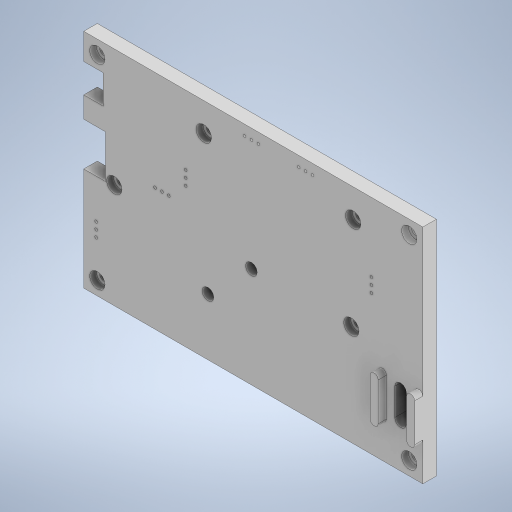
# Autodesk Inventor part: base_main
Saved by Autodesk Inventor 2024.2 (Build 282272000, 272)
## iProperties
Created: 2021-12-13
Part Number: base_main
Material: Generic
Document SubType Name: Modeling
Designer: magoo
Density: 1 g/cm^3
Appearance: Default
Description: 3D printing model
Author: magoo
Autodesk Inventor part; units mm, degrees
ref_plane "YZ Plane" through (0, 0, 0) normal (1, 0, 0) x (0, 1, 0)
ref_plane "XZ Plane" through (0, 0, 0) normal (0, 1, 0) x (-1, 0, 0)
ref_plane "XY Plane" through (0, 0, 0) normal (0, 0, 1) x (1, 0, 0)
sketch "Sketch1" plane through (0, 0, 0) normal (0, 0, 1) x (1, 0, 0)
  line L0 (65, -35) -> (-65, -35)
  line L1 (-65, -35) -> (-65, 35)
  line L2 (-65, 35) -> (65, 35)
  line L3 (65, 35) -> (65, -35)
  line L4 (65, -35) -> (-65, 35) construction
  line L5 (-65, -35) -> (65, 35) construction
  line L6 (56.8, -15) -> (56.8, -25) construction
  line L7 (54.65, -15) -> (54.65, -25)
  line L8 (58.95, -25) -> (58.95, -15)
  arc A0 (58.95, -15) -> (54.65, -15) centre (56.8, -15) ccw
  arc A1 (54.65, -25) -> (58.95, -25) centre (56.8, -25) ccw
  line L9 (62, -13) -> (65, -13)
  line L10 (65, -13) -> (65, -27)
  line L11 (65, -27) -> (62, -27)
  line L12 (62, -27) -> (62, -13)
  line L13 (62, -13) -> (65, -27) construction
  line L14 (65, -13) -> (62, -27) construction
  line L15 (56.8, -20) -> (63.5, -20) construction
  line L16 (48.6, -13) -> (51.6, -13)
  line L17 (51.6, -13) -> (51.6, -27)
  line L18 (51.6, -27) -> (48.6, -27)
  line L19 (48.6, -27) -> (48.6, -13)
  line L20 (48.6, -13) -> (51.6, -27) construction
  line L21 (51.6, -13) -> (48.6, -27) construction
  line L22 (50.1, -20) -> (56.8, -20) construction
  circle A2 centre (56.8, -20) radius 0.5
  line L23 (56.8, -20) -> (-65, -20)
  line L24 (-60, 35) -> (-60, -35)
  line L25 (-65, 35) -> (65, 35)
  line L26 (65, 35) -> (65, 41)
  line L27 (65, 41) -> (-65, 41)
  line L28 (-65, 41) -> (-65, 35)
  line L29 (-60, 35) -> (-60, 41)
  circle A3 centre (50.1, -13) radius 1.5
  circle A4 centre (63.5, -13) radius 1.5
  circle A5 centre (50.1, -27) radius 1.5
  circle A6 centre (63.5, -27) radius 1.5
  line L30 (-65, -35) -> (-65, -41)
  line L31 (-65, -41) -> (65, -41)
  line L32 (65, -41) -> (65, -35)
  line L33 (-60, -35) -> (-60, -41)
  point P0 (0, 0)
  point P1 (65, -27)
  point P2 (65, -13)
  point P3 (65, -13)
  dimension "d0" = 70
  dimension "d1" = 130
  dimension "d2" = 10
  dimension "d3" = 4.3
  dimension "d4" = 14
  dimension "d5" = 3
  dimension "d6" = 14
  dimension "d7" = 3
  dimension "d10" = 8
  dimension "d11" = 0
  dimension "d16" = 1
  dimension "d20" = 5.2
  dimension "d21" = 5.2
  dimension "d22" = 5
  dimension "d23" = 6
  dimension "d26" = 125
  dimension "d27" = 76
  dimension "d122" = 6
  constraints: 70 end point, 11 midpoint, 9 parallel, 9 perpendicular, 6 horizontal, 6 point on line, 4 point on circle, 4 tangent, 3 centre point, 3 coincident, 2 vertical, 12 other
  measures "d0" distance of L2.end L0.start
  measures "d1" distance of L1.end L2.end
  measures "d2" distance of L6.start L6.end
  measures "d3" distance between parallel lines of L8 L7
  measures "d4" distance of L9.end L10.end
  measures "d5" distance of L10.end L11.end
  measures "d6" distance of L18.end L16.start
  measures "d7" distance of L17.end L18.end
  measures "d10" distance from line of L0 point (63.5, -27)
  measures "d11" distance between parallel lines of L3 L10
  measures "d16" diameter of A2
  measures "d20" distance between parallel lines of L12 L6
  measures "d21" distance between parallel lines of L17 L6
  measures "d22" distance between parallel lines of L1 L24
  measures "d23" distance of L27.end L1.end
  measures "d26" distance between parallel lines of L24 L3
  measures "d27" distance between parallel lines of L0 L27
  measures "d122" distance of L31.end L0.start
extrude "Extrusion1" add sketch "Sketch1" against normal blind 5 contours L32 L31 L33 L0 | L19 A3 L17 L23 | L23 L17 A5 L19 | L0 L24 L2 L3 A4 L12 A6 | A6 L12 A4 L3 | A6 L11 | L11 A6 | A4 L9 | L9 A4 | L29 L27 L26 L2 | A5 L18 | L18 A5 | A3 L16 | L16 A3
extrude "Extrusion2" add sketch "Sketch1" along normal blind 3 contours L19 A3 L17 L23 | L23 L17 A5 L19 | A6 L12 A4 L3 | A6 L11 | L11 A6 | A4 L9 | L9 A4 | A5 L18 | L18 A5 | A3 L16 | L16 A3
sketch "Sketch4" plane through (0, 0, -5) normal (0, 0, -1) x (-1, 0, 0)
  circle A0 centre (55.4192, -22.54) radius 0.2032 construction
  circle A1 centre (55.4192, -20) radius 0.2032 construction
  circle A2 centre (55.4192, -17.46) radius 0.2032 construction
  circle A3 centre (33.74, 4.2192) radius 0.2032 construction
  circle A4 centre (31.2, 4.2192) radius 0.2032 construction
  circle A5 centre (28.66, 4.2192) radius 0.2032 construction
  circle A6 centre (22.4192, 10.46) radius 0.2032 construction
  circle A7 centre (22.4192, 13) radius 0.2032 construction
  circle A8 centre (22.4192, 15.54) radius 0.2032 construction
  circle A9 centre (-46.0192, 10.46) radius 0.2032 construction
  circle A10 centre (-46.0192, 13) radius 0.2032 construction
  circle A11 centre (-46.0192, 15.54) radius 0.2032 construction
  circle A12 centre (-24.34, 37.2192) radius 0.2032 construction
  circle A13 centre (-21.8, 37.2192) radius 0.2032 construction
  circle A14 centre (-19.26, 37.2192) radius 0.2032 construction
  circle A15 centre (-4.34, 37.2192) radius 0.2032 construction
  circle A16 centre (-1.8, 37.2192) radius 0.2032 construction
  circle A17 centre (0.74, 37.2192) radius 0.2032 construction
  circle A18 centre (55, 36) radius 1.6
  arc A19 (-26.0469, -12.3763) -> (-29.4237, -15.7531) centre (-28.7, -13.1) ccw construction
  arc A20 (-29.4237, -24.2469) -> (-26.0469, -27.6237) centre (-28.7, -26.9) ccw construction
  line L0 (-48.6, -13) -> (-48.6, -27) construction
  circle A21 centre (-56.8, -20) radius 2.3368 construction
  line L1 (-28.7, -26.9) -> (-28.7, -13.1) construction
  line L2 (-56.8, -20) -> (-48.6, -20) construction
  line L3 (-48.6, -20) -> (-28.7, -20) construction
  line L4 (-38.65, -20) -> (-38.65, -36) construction
  line L5 (60, -41) -> (60, 41) construction
  line L6 (60, 36) -> (-65, 36) construction
  line L7 (55, -4) -> (55, 36) construction
  line L8 (-38.65, -20) -> (-38.65, 36) construction
  line L9 (60, 41) -> (-65, 41) construction
  circle A22 centre (-1.8, -4) radius 2.15 projected
  circle A23 centre (14.2, -20) radius 2.15 projected
  line L10 (-1.8, -4) -> (60, -4) construction
  circle A24 centre (55.4192, -22.54) radius 0.5
  circle A25 centre (55.4192, -20) radius 0.5
  circle A26 centre (55.4192, -17.46) radius 0.5
  circle A27 centre (33.74, 4.2192) radius 0.5
  circle A28 centre (31.2, 4.2192) radius 0.5
  circle A29 centre (28.66, 4.2192) radius 0.5
  circle A30 centre (-46.0192, 10.46) radius 0.5
  circle A31 centre (-46.0192, 13) radius 0.5
  circle A32 centre (-46.0192, 15.54) radius 0.5
  circle A33 centre (0.74, 37.2192) radius 0.5
  circle A34 centre (-1.8, 37.2192) radius 0.5
  circle A35 centre (-4.34, 37.2192) radius 0.5
  circle A36 centre (-19.26, 37.2192) radius 0.5
  circle A37 centre (-21.8, 37.2192) radius 0.5
  circle A38 centre (-24.34, 37.2192) radius 0.5
  line L11 (55, -4) -> (55, -35) construction
  line L12 (60, 41) -> (60, -41) construction
  line L13 (60, -36) -> (-65, -36) construction
  circle A39 centre (55, -36) radius 1.6
  line L14 (-60, 41) -> (-60, -35) construction
  circle A40 centre (-60, 36) radius 1.6
  line L15 (22.4192, 13) -> (55, 13) construction
  line L16 (-1.8, -4) -> (-38.65, -4) construction
  circle A41 centre (-38.65, -4) radius 1.6
  line L17 (22.4192, 13) -> (-65, 13) construction
  line L18 (55.4192, -22.54) -> (28.66, -22.54) construction
  line L19 (28.66, -22.54) -> (28.66, 4.2192) construction
  line L20 (28.66, 4.2192) -> (55.4192, 4.2192) construction
  line L21 (55.4192, 4.2192) -> (55.4192, -22.54) construction
  line L22 (-4.34, 37.2192) -> (22.4192, 37.2192) construction
  line L23 (22.4192, 37.2192) -> (22.4192, 10.46) construction
  line L24 (22.4192, 10.46) -> (-4.34, 10.46) construction
  line L25 (-4.34, 10.46) -> (-4.34, 37.2192) construction
  line L26 (-19.26, 37.2192) -> (-46.0192, 37.2192) construction
  line L27 (-46.0192, 37.2192) -> (-46.0192, 10.46) construction
  line L28 (-46.0192, 10.46) -> (-19.26, 10.46) construction
  line L29 (-19.26, 10.46) -> (-19.26, 37.2192) construction
  line L30 (-32.6396, 37.2192) -> (-32.6396, 10.46) construction
  line L31 (-32.6396, 23.8396) -> (-46.0192, 23.8396) construction
  line L32 (-39.3294, 23.8396) -> (-39.3294, 37.2192) construction
  circle A42 centre (-39.3294, 30.5294) radius 1.6
  line L33 (9.0396, 37.2192) -> (9.0396, 10.46) construction
  line L34 (9.0396, 23.8396) -> (22.4192, 23.8396) construction
  line L35 (15.7294, 23.8396) -> (15.7294, 37.2192) construction
  circle A43 centre (15.7294, 30.5294) radius 1.6
  line L36 (42.0396, 4.2192) -> (42.0396, -22.54) construction
  line L37 (42.0396, -9.1604) -> (55.4192, -9.1604) construction
  line L38 (48.7294, -9.1604) -> (48.7294, 4.2192) construction
  circle A44 centre (48.7294, -2.4706) radius 1.6
  circle A45 centre (22.4192, 10.46) radius 0.2032 construction
  circle A46 centre (22.4192, 13) radius 0.2032 construction
  circle A47 centre (22.4192, 15.54) radius 0.2032 construction
  circle A48 centre (22.4192, 15.54) radius 0.5
  circle A49 centre (22.4192, 13) radius 0.5
  circle A50 centre (22.4192, 10.46) radius 0.5
  line L39 (-65, -41) -> (60, -41) projected
  line L40 (-65, 41) -> (-65, -41) projected
  circle A51 centre (-60, -36) radius 1.6
  point P0 (0, 0)
  dimension "d29" = 3.2
  dimension "d32" = 5
  dimension "d33" = 5
  dimension "d36" = 1
  dimension "d37" = 1
  dimension "d38" = 1
  dimension "d39" = 1
  dimension "d40" = 1
  dimension "d41" = 1
  dimension "d42" = 1
  dimension "d43" = 1
  dimension "d44" = 1
  dimension "d45" = 1
  dimension "d46" = 1
  dimension "d47" = 1
  dimension "d48" = 1
  dimension "d49" = 1
  dimension "d50" = 1
  dimension "d54" = 3.2
  dimension "d57" = 3.2
  dimension "d59" = 3.2
  dimension "d61" = 3.2
  dimension "d62" = 3.2
  dimension "d63" = 3.2
  dimension "d64" = 1
  dimension "d65" = 1
  dimension "d66" = 1
  dimension "d123" = 5
  dimension "d124" = 5
  dimension "d135" = 3.2
  constraints: 70 end point, 26 centre point, 21 midpoint, 20 coincident, 20 point on line, 13 perpendicular, 6 parallel, 5 horizontal, 3 vertical
  measures "d29" diameter of A18
  measures "d32" distance between parallel lines of L9 L6
  measures "d33" distance between parallel lines of L5 L7
  measures "d36" diameter of A24
  measures "d37" diameter of A25
  measures "d38" diameter of A26
  measures "d39" diameter of A27
  measures "d40" diameter of A28
  measures "d41" diameter of A29
  measures "d42" diameter of A30
  measures "d43" diameter of A31
  measures "d44" diameter of A32
  measures "d45" diameter of A33
  measures "d46" diameter of A34
  measures "d47" diameter of A35
  measures "d48" diameter of A36
  measures "d49" diameter of A37
  measures "d50" diameter of A38
  measures "d54" diameter of A39
  measures "d57" diameter of A40
  measures "d59" diameter of A41
  measures "d61" diameter of A42
  measures "d62" diameter of A43
  measures "d63" diameter of A44
  measures "d64" diameter of A48
  measures "d65" diameter of A49
  measures "d66" diameter of A50
  measures "d123" distance between parallel lines of L39 L13
  measures "d124" distance between parallel lines of L40 L14
  measures "d135" diameter of A51
extrude "Extrusion6" cut sketch "Sketch4" against normal up to next
sketch "Sketch7" plane through (0, 0, 0) normal (0, 0, 1) x (1, 0, 0)
  circle A0 centre (-15.7294, 30.5294) radius 1.6 projected
  circle A1 centre (-55.4192, -17.46) radius 0.5 projected
  circle A2 centre (-22.4192, 10.46) radius 0.5 projected
  circle A3 centre (1.8, 37.2192) radius 0.5 projected
  circle A4 centre (24.34, 37.2192) radius 0.5 projected
  circle A5 centre (-14.2, -20) radius 2.15 projected
  circle A6 centre (46.0192, 15.54) radius 0.5 projected
  circle A7 centre (21.8, 37.2192) radius 0.5 projected
  circle A8 centre (-0.74, 37.2192) radius 0.5 projected
  circle A9 centre (-28.66, 4.2192) radius 0.5 projected
  circle A10 centre (-55.4192, -20) radius 0.5 projected
  circle A11 centre (-48.7294, -2.4706) radius 1.6 projected
  circle A12 centre (39.3294, 30.5294) radius 1.6 projected
  circle A13 centre (38.65, -4) radius 1.6 projected
  circle A14 centre (-55, 36) radius 1.6 projected
  circle A15 centre (-33.74, 4.2192) radius 0.5 projected
  circle A16 centre (-22.4192, 13) radius 0.5 projected
  circle A17 centre (4.34, 37.2192) radius 0.5 projected
  circle A18 centre (46.0192, 10.46) radius 0.5 projected
  circle A19 centre (1.8, -4) radius 2.15 projected
  circle A20 centre (46.0192, 13) radius 0.5 projected
  circle A21 centre (19.26, 37.2192) radius 0.5 projected
  circle A22 centre (-22.4192, 15.54) radius 0.5 projected
  circle A23 centre (-31.2, 4.2192) radius 0.5 projected
  circle A24 centre (-55.4192, -22.54) radius 0.5 projected
  circle A25 centre (-55, -36) radius 1.6 projected
  circle A26 centre (60, 36) radius 1.6 projected
  line L0 (54.65, -15) -> (54.65, -25) projected
  arc A27 (54.65, -25) -> (58.95, -25) centre (56.8, -25) ccw projected
  line L1 (58.95, -25) -> (58.95, -15) projected
  arc A28 (58.95, -15) -> (54.65, -15) centre (56.8, -15) ccw projected
  line L2 (-60, -41) -> (-60, 41) projected
  line L3 (-60, 41) -> (65, 41) projected
  circle A29 centre (1.8, -4) radius 4
  circle A30 centre (-14.2, -20) radius 4
  line L4 (52.8, -25) -> (52.8, -15)
  arc A31 (60.8, -15) -> (52.8, -15) centre (56.8, -15) ccw
  line L5 (60.8, -15) -> (60.8, -25)
  arc A32 (52.8, -25) -> (60.8, -25) centre (56.8, -25) ccw
  line L6 (65, 41) -> (65, -41) projected
  line L7 (65, -41) -> (-60, -41) projected
  point P0 (0, 0)
  dimension "d69" = 1.85
  dimension "d70" = 1.85
  dimension "d71" = 1.85
  constraints: 4 centre point, 4 end point, 4 point on circle, 3 other
  measures "d69" radial gap between concentric circles of A19 A29
  measures "d70" radial gap between concentric circles of A5 A30
  measures "d71" distance between parallel lines of L0 L4
sketch "Sketch8" plane through (0, 0, 0) normal (0, 0, 1) x (1, 0, 0)
  circle A0 centre (-48.7294, -2.4706) radius 1.6 construction
  circle A1 centre (-55, 36) radius 1.6 construction
  circle A2 centre (-15.7294, 30.5294) radius 1.6 construction
  circle A3 centre (39.3294, 30.5294) radius 1.6 construction
  circle A4 centre (60, 36) radius 1.6 construction
  circle A5 centre (38.65, -4) radius 1.6 construction
  circle A6 centre (-55, -36) radius 1.6 construction
  circle A7 centre (-55, 36) radius 1.6 projected
  circle A8 centre (-55, 36) radius 2.85
  circle A9 centre (-15.7294, 30.5294) radius 1.6 projected
  circle A10 centre (-15.7294, 30.5294) radius 2.85
  circle A11 centre (39.3294, 30.5294) radius 1.6 projected
  circle A12 centre (39.3294, 30.5294) radius 2.85
  circle A13 centre (60, 36) radius 1.6 projected
  circle A14 centre (60, 36) radius 2.85
  circle A15 centre (-48.7294, -2.4706) radius 2.85
  circle A16 centre (38.65, -4) radius 1.6 projected
  circle A17 centre (38.65, -4) radius 2.85
  circle A18 centre (-55, -36) radius 2.85
  circle A19 centre (60, -36) radius 1.6 projected
  circle A20 centre (60, -36) radius 2.85
  point P0 (0, 0)
  point P1 (0.2167, -2.5455)
  point P2 (0.2167, -5.4545)
  dimension "d72" = 5.7
  dimension "d73" = 5.7
  dimension "d74" = 5.7
  dimension "d75" = 5.7
  dimension "d76" = 5.7
  dimension "d77" = 5.7
  dimension "d78" = 5.7
  dimension "d136" = 5.7
  constraints: 8 centre point, 8 coincident, 2 other
  measures "d72" diameter of A8
  measures "d73" diameter of A10
  measures "d74" diameter of A12
  measures "d75" diameter of A14
  measures "d76" diameter of A15
  measures "d77" diameter of A17
  measures "d78" diameter of A18
  measures "d136" diameter of A20
extrude "Extrusion7" cut sketch "Sketch8" against normal blind 2.5 contours A8 | A10 | A12 | A14 | A15 | A16 | A17 | A18 | A20
sketch "Sketch12" plane through (0, 0, 0) normal (0, 0, 1) x (1, 0, 0)
  line L0 (-60, 31.36) -> (-52.8, 31.36)
  line L1 (-52.8, 31.36) -> (-52.8, 20.71)
  line L2 (-52.8, 20.71) -> (-60, 20.71)
  line L3 (-60, 20.71) -> (-60, 31.36)
  line L4 (-58.2, 26.76) -> (-58.2, 26.56) construction
  line L5 (-58.2, 25.51) -> (-58.2, 25.31) construction
  line L6 (-54.75, 21.21) -> (-55.25, 21.21) construction
  line L7 (-54.75, 30.86) -> (-55.25, 30.86) construction
  line L8 (-53.3, 25.586) -> (-53.3, 26.484) construction
  line L9 (-60, 12.432) -> (-52.507, 12.432) construction
  line L10 (-52.507, 12.432) -> (-52.507, 9.9) construction
  line L11 (-52.507, 9.9) -> (-60, 9.9) construction
  line L12 (-60, 0.1) -> (-52.507, 0.1) construction
  line L13 (-52.507, 0.1) -> (-52.507, -2.442) construction
  line L14 (-52.507, -2.442) -> (-60, -2.442) construction
  line L15 (-60, 12.932) -> (-52.007, 12.932)
  line L16 (-52.007, 12.932) -> (-52.007, -2.942)
  line L17 (-52.007, -2.942) -> (-60, -2.942)
  line L18 (-60, -2.942) -> (-60, 12.932)
  line L19 (-60, 41) -> (-60, -41) projected
  point P0 (0, 0)
  point P1 (-55, 30.86)
  point P2 (-55, 21.21)
  point P3 (-53.3, 26.035)
  point P4 (-58.2, 26.66)
  point P5 (-52.507, 11.166)
  point P6 (-56.2535, 12.432)
  point P7 (-56.2535, -2.442)
  dimension "d148" = 0.5
  dimension "d149" = 0.5
  dimension "d151" = 0.5
  dimension "d152" = 0.5
  dimension "d153" = 0.5
  dimension "d154" = 0
  dimension "d155" = 0
  dimension "d158" = 0.5
  constraints: 16 end point, 7 midpoint, 4 parallel, 2 horizontal, 2 perpendicular
  measures "d148" distance from line of L2 point (-55, 21.21)
  measures "d149" distance from line of L1 point (-53.3, 26.035)
  measures "d151" distance from line of L16 point (-52.507, 11.166)
  measures "d152" distance from line of L15 point (-56.253, 12.432)
  measures "d153" distance from line of L17 point (-56.253, -2.442)
  measures "d154" distance between parallel lines of L18 L19
  measures "d155" distance between parallel lines of L3 L19
  measures "d158" distance from line of L0 point (-55, 30.86)
extrude "Extrusion12" cut sketch "Sketch12" against normal through all
body "Solid1"
